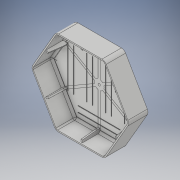
# Autodesk Inventor part: Base v5 - 175
Saved by Autodesk Inventor 2019 (Build 230136000, 136)
## iProperties
Created: 2021-07-14
Part Number: Base v5 - 175
Material: Generic
Document SubType Name: Modeling
Designer: Lix
Density: 1 g/cm^3
Appearance: Default
Author: Lix
## iProperties of the stored document Base v6 - 175 - thicker wall_3DPrint.ipt
Created: 2021-08-11
Part Number: Base v6 - 175 - thicker wall_3DPrint
Material: Generic
Document SubType Name: Modeling
Designer: Lix
Density: 1 g/cm^3
Appearance: Default
Author: Lix
Autodesk Inventor part; units mm, degrees
sketch "Sketch1" plane through (0, 0, 0) normal (0, 0, 1) x (1, 0, 0)
  line L0 (50.5181, -87.5) -> (-50.5181, -87.5)
  line L1 (-50.5181, -87.5) -> (-101.0363, 0)
  line L2 (-101.0363, 0) -> (-50.5181, 87.5)
  line L3 (-50.5181, 87.5) -> (50.5181, 87.5)
  line L4 (50.5181, 87.5) -> (101.0363, 0)
  line L5 (101.0363, 0) -> (50.5181, -87.5)
  point P0 (0, 0)
  point P1 (0, 0)
  point P2 (0, 0)
  dimension "d0" = 175
  constraints: 12 end point, 2 coincident, 1 horizontal, 13 other
  measures "d0" distance between parallel lines of L5 L2
extrude "Extrusion1" add sketch "Sketch1" along normal blind 40
shell "Shell1" thickness 2.5 removed faces 1 at (16.8394, -29.1667, 40) ; own thickness 1 on faces at (16.8394, -29.1667, 0)
sketch "Sketch11" plane through (-49.0748, -85, 1) normal (0, 0, 1) x (1, 0, 0)
  line L0 (-9.4252, 85) -> (107.5748, 85) construction
  line L1 (6.7369, 14.5052) -> (91.4127, 14.5052)
  line L2 (91.4127, 14.5052) -> (91.4127, 25.4948)
  line L3 (91.4127, 25.4948) -> (6.7369, 25.4948)
  line L4 (6.7369, 25.4948) -> (6.7369, 14.5052)
  line L5 (6.7369, 14.5052) -> (91.4127, 25.4948) construction
  line L6 (91.4127, 14.5052) -> (6.7369, 25.4948) construction
  line L7 (49.0748, 20) -> (49.0748, 150) construction
  line L8 (6.7369, 144.5052) -> (91.4127, 144.5052)
  line L9 (91.4127, 144.5052) -> (91.4127, 155.4948)
  line L10 (91.4127, 155.4948) -> (6.7369, 155.4948)
  line L11 (6.7369, 155.4948) -> (6.7369, 144.5052)
  line L12 (6.7369, 144.5052) -> (91.4127, 155.4948) construction
  line L13 (91.4127, 144.5052) -> (6.7369, 155.4948) construction
  line L14 (5.7369, 156.4948) -> (92.4127, 156.4948)
  line L15 (92.4127, 156.4948) -> (92.4127, 143.5052)
  line L16 (92.4127, 143.5052) -> (5.7369, 143.5052)
  line L17 (5.7369, 143.5052) -> (5.7369, 156.4948)
  line L18 (92.4127, 13.5052) -> (5.7369, 13.5052)
  line L19 (5.7369, 13.5052) -> (5.7369, 26.4948)
  line L20 (5.7369, 26.4948) -> (92.4127, 26.4948)
  line L21 (92.4127, 26.4948) -> (92.4127, 13.5052)
  line L22 (92.4127, 155.5) -> (5.7369, 155.5)
  line L23 (5.7369, 155.5) -> (5.7369, 144.5)
  line L24 (5.7369, 144.5) -> (92.4127, 144.5)
  line L25 (92.4127, 144.5) -> (92.4127, 155.5)
  line L26 (92.4127, 25.5) -> (5.7369, 25.5)
  line L27 (5.7369, 25.5) -> (5.7369, 14.5)
  line L28 (5.7369, 14.5) -> (92.4127, 14.5)
  line L29 (92.4127, 14.5) -> (92.4127, 25.5)
  line L30 (-3.9252, 128.5) -> (-3.9252, 41.5)
  line L31 (-14.9252, 41.5) -> (-14.9252, 128.5)
  line L32 (-14.9252, 128.5) -> (-3.9252, 41.5) construction
  line L33 (-3.9252, 128.5) -> (-14.9252, 41.5) construction
  line L34 (147.2243, 85) -> (98.1495, 0) projected
  line L35 (0, 170) -> (98.1495, 0) construction
  line L36 (-14.9252, 128.5) -> (-15.9252, 128.5)
  line L37 (-15.9252, 128.5) -> (-15.9252, 41.5)
  line L38 (-15.9252, 41.5) -> (-14.9252, 41.5)
  line L39 (-14.9252, 41.5) -> (-14.9252, 128.5)
  line L40 (-3.9252, 41.5) -> (-2.9252, 41.5)
  line L41 (-2.9252, 41.5) -> (-2.9252, 128.5)
  line L42 (-2.9252, 128.5) -> (-3.9252, 128.5)
  line L43 (-3.9252, 128.5) -> (-3.9252, 41.5)
  line L44 (36.0748, 41.5) -> (36.0748, 128.5)
  line L45 (35.0748, 41.5) -> (36.0748, 41.5)
  line L46 (36.0748, 128.5) -> (35.0748, 128.5)
  line L47 (35.0748, 128.5) -> (35.0748, 41.5)
  line L48 (35.0748, 128.5) -> (35.0748, 41.5)
  line L49 (24.0748, 41.5) -> (24.0748, 128.5)
  line L50 (24.0748, 128.5) -> (35.0748, 41.5) construction
  line L51 (24.0748, 41.5) -> (24.0748, 128.5)
  line L52 (24.0748, 128.5) -> (23.0748, 128.5)
  line L53 (23.0748, 128.5) -> (23.0748, 41.5)
  line L54 (23.0748, 41.5) -> (24.0748, 41.5)
  line L55 (35.0748, 128.5) -> (24.0748, 41.5) construction
  line L56 (75.0748, 41.5) -> (75.0748, 128.5)
  line L57 (74.0748, 41.5) -> (75.0748, 41.5)
  line L58 (75.0748, 128.5) -> (74.0748, 128.5)
  line L59 (74.0748, 128.5) -> (74.0748, 41.5)
  line L60 (74.0748, 128.5) -> (74.0748, 41.5)
  line L61 (63.0748, 41.5) -> (63.0748, 128.5)
  line L62 (63.0748, 128.5) -> (74.0748, 41.5) construction
  line L63 (63.0748, 41.5) -> (63.0748, 128.5)
  line L64 (63.0748, 128.5) -> (62.0748, 128.5)
  line L65 (62.0748, 128.5) -> (62.0748, 41.5)
  line L66 (62.0748, 41.5) -> (63.0748, 41.5)
  line L67 (74.0748, 128.5) -> (63.0748, 41.5) construction
  line L68 (114.0748, 41.5) -> (114.0748, 128.5)
  line L69 (113.0748, 41.5) -> (114.0748, 41.5)
  line L70 (114.0748, 128.5) -> (113.0748, 128.5)
  line L71 (113.0748, 128.5) -> (113.0748, 41.5)
  line L72 (113.0748, 128.5) -> (113.0748, 41.5)
  line L73 (102.0748, 41.5) -> (102.0748, 128.5)
  line L74 (102.0748, 128.5) -> (113.0748, 41.5) construction
  line L75 (102.0748, 41.5) -> (102.0748, 128.5)
  line L76 (102.0748, 128.5) -> (101.0748, 128.5)
  line L77 (101.0748, 128.5) -> (101.0748, 41.5)
  line L78 (101.0748, 41.5) -> (102.0748, 41.5)
  line L79 (113.0748, 128.5) -> (102.0748, 41.5) construction
  circle A0 centre (-41.4556, 85) radius 0.5
  circle A1 centre (-38.4556, 85) radius 0.5
  point P0 (49.0748, 85)
  point P1 (29.5748, 85)
  point P2 (68.5748, 85)
  point P3 (107.5748, 85)
  dimension "d147" = 130
  dimension "d151" = 1
  dimension "d156" = 1
  dimension "d157" = 11
  dimension "d158" = 87
  dimension "d167" = 117
  dimension "d168" = 1
  dimension "d169" = 87
  dimension "d170" = 1
  dimension "d171" = 87
  dimension "d174" = 39
  dimension "d179" = 1
  dimension "d180" = 1
  dimension "d181" = 3
  constraints: 158 end point, 17 parallel, 15 midpoint, 8 horizontal, 8 perpendicular, 4 point on line, 2 centre point, 2 equal length, 1 vertical, 75 other
  measures "d147" distance of L7.start L7.end
  measures "d151" distance between parallel lines of L10 L14
  measures "d156" distance between parallel lines of L1 L18
  measures "d157" distance of L30.end L31.start
  measures "d158" distance of L30.start L30.end
  measures "d167" distance of L0.start L0.end
  measures "d168" distance of L38.end L37.end
  measures "d169" distance of L37.end L36.end
  measures "d170" distance of L42.end L41.end
  measures "d171" distance of L41.end L40.end
  measures "d174" distance of L0.start point (29.575, 85)
  measures "d179" diameter of A0
  measures "d180" diameter of A1
  measures "d181" distance of A1.centre A0.centre
extrude "Extrusion9" add sketch "Sketch11" along normal blind 0.5 contours L14 L15 L22 L17 | L24 L15 L16 L17 | L18 L19 L28 L21 | L26 L19 L20 L21 | L42 L41 L40 L30 | L38 L37 L36 L31 | L45 L47 L46 L44 | L54 L53 L52 L49 | L57 L59 L58 L56 | L66 L65 L64 L61 | L69 L71 L70 L68 | L78 L77 L76 L73 | A0 | A1
ref_plane "Work Plane1" through (-25.2591, 43.75, 40) normal (0.8660254, 0.5, 0) x (0, 0, -1)
ref_plane "Work Plane2" through (-50.5181, 0, 0) normal (0, 1, 0) x (1, 0, 0)
ref_plane "Work Plane3" through (-25.2591, -43.75, 0) normal (-0.8660254, 0.5, 0) x (0, 0, 1)
sketch "Sketch12" plane through (-49.0748, -85, 1) normal (0, 0, 1) x (1, 0, 0)
  line L0 (98.1495, 0) -> (0, 0) projected
  line L1 (147.2243, 85) -> (98.1495, 0) projected
  line L2 (98.1495, 170) -> (147.2243, 85) projected
  line L3 (0, 170) -> (98.1495, 170) projected
  line L4 (-49.0748, 85) -> (0, 170) projected
  line L5 (0, 0) -> (-49.0748, 85) projected
  point P0 (49.0748, 85)
sketch "Sketch4" plane through (-49.0748, -85, 1) normal (0, 0, 1) x (1, 0, 0)
  line L0 (98.1495, 0) -> (0, 0) projected
  line L1 (147.2243, 85) -> (98.1495, 0) projected
  line L2 (98.1495, 170) -> (147.2243, 85) projected
  line L3 (0, 170) -> (98.1495, 170) projected
  line L4 (-49.0748, 85) -> (0, 170) projected
  line L5 (0, 0) -> (-49.0748, 85) projected
  line L6 (-18.9944, 127.1007) -> (2.8868, 165)
  line L7 (2.8868, 165) -> (46.6491, 165)
  line L8 (98.1495, 170) -> (0, 0) construction
  arc A0 (46.6491, 94.7014) -> (41.886, 91.9514) centre (49.0748, 85) ccw
  line L9 (-18.9944, 127.1007) -> (41.886, 91.9514)
  line L10 (46.6491, 165) -> (46.6491, 94.7014)
  circle A1 centre (49.0748, 85) radius 2.5
  arc A2 (39.4603, 87.75) -> (39.4603, 82.25) centre (49.0748, 85) ccw
  line L11 (-21.4201, 122.8993) -> (39.4603, 87.75)
  line L12 (-21.4201, 47.1007) -> (39.4603, 82.25)
  line L13 (-21.4201, 47.1007) -> (-43.3013, 85)
  line L14 (-43.3013, 85) -> (-21.4201, 122.8993)
  arc A3 (41.886, 78.0486) -> (46.6491, 75.2986) centre (49.0748, 85) ccw
  line L15 (-18.9944, 42.8993) -> (41.886, 78.0486)
  line L16 (46.6491, 5) -> (46.6491, 75.2986)
  line L17 (46.6491, 5) -> (2.8868, 5)
  line L18 (2.8868, 5) -> (-18.9944, 42.8993)
  arc A4 (51.5004, 75.2986) -> (56.2636, 78.0486) centre (49.0748, 85) ccw
  line L19 (51.5004, 5) -> (51.5004, 75.2986)
  line L20 (117.144, 42.8993) -> (56.2636, 78.0486)
  line L21 (117.144, 42.8993) -> (95.2628, 5)
  line L22 (95.2628, 5) -> (51.5004, 5)
  arc A5 (58.6892, 82.25) -> (58.6892, 87.75) centre (49.0748, 85) ccw
  line L23 (119.5696, 47.1007) -> (58.6892, 82.25)
  line L24 (119.5696, 122.8993) -> (58.6892, 87.75)
  line L25 (119.5696, 122.8993) -> (141.4508, 85)
  line L26 (141.4508, 85) -> (119.5696, 47.1007)
  arc A6 (56.2636, 91.9514) -> (51.5004, 94.7014) centre (49.0748, 85) ccw
  line L27 (117.144, 127.1007) -> (56.2636, 91.9514)
  line L28 (51.5004, 165) -> (51.5004, 94.7014)
  line L29 (51.5004, 165) -> (95.2628, 165)
  line L30 (95.2628, 165) -> (117.144, 127.1007)
  point P0 (-49.0748, 85)
  point P1 (0, 0)
  point P2 (98.1495, 0)
  point P3 (147.2243, 85)
  point P4 (98.1495, 170)
  dimension "d37" = 5
  dimension "d44" = 10
  dimension "d45" = 60
  dimension "d46" = 90
  dimension "d47" = 90
  dimension "d52" = 5.5
  dimension "d55" = 5
  dimension "d72" = 360
  constraints: 50 end point, 12 point on circle, 7 centre point, 2 coincident, 2 equal length, 1 midpoint, 73 other
  measures "d37" distance between parallel lines of L3 L7
  measures "d44" radius of A0
  measures "d45" angle of L10 L9
  measures "d46" angle of L9 L6
  measures "d47" angle of L10 L7
  measures "d52" distance of L10.end L9.end
  measures "d55" diameter of A1
extrude "Extrusion5" cut sketch "Sketch4" against normal blind 0.01 contours L6 L7 L10 A0 L9 | A1 | A2 L12 L13 L14 L11 | A3 L16 L17 L18 L15 | A4 L20 L21 L22 L19 | A5 L24 L25 L26 L23 | A6 L28 L29 L30 L27
sketch "Sketch8" plane through (-49.0748, -85, 1) normal (0, 0, 1) x (1, 0, 0)
  line L0 (98.1495, 0) -> (0, 0) projected
  line L1 (147.2243, 85) -> (98.1495, 0) projected
  line L2 (98.1495, 170) -> (147.2243, 85) projected
  line L3 (0, 170) -> (98.1495, 170) projected
  line L4 (-49.0748, 85) -> (0, 170) projected
  line L5 (0, 0) -> (-49.0748, 85) projected
  line L6 (47.5748, 162) -> (50.5748, 162)
  line L7 (50.5748, 162) -> (50.5748, 170)
  line L8 (50.5748, 170) -> (47.5748, 170)
  line L9 (47.5748, 170) -> (47.5748, 162)
  line L10 (0, 170) -> (98.1495, 170) projected
  line L11 (49.0748, 86) -> (49.0748, 170)
  point P0 (49.0748, 85)
  dimension "d57" = 3
  dimension "d58" = 8
  constraints: 10 end point, 2 midpoint, 2 parallel, 1 coincident, 1 collinear, 1 horizontal, 1 perpendicular, 1 vertical
  measures "d57" distance of L6.start L6.end
  measures "d58" distance of L6.end L7.end
extrude "Extrusion6" add sketch "Sketch8" along normal blind 36 contours L7 L6 L11 L3 | L3 L11 L6 L9
sketch "Sketch9" plane through (1.5, 77, 1) normal (1, 0, 0) x (0, 0, -1)
  line L0 (0, 0) -> (0, 8) projected
  line L1 (0, 0) -> (-36, 0) projected
  line L2 (-36, 8) -> (-36, 0) projected
  line L3 (0, 8) -> (-36, 8) projected
  line L4 (-36, 8) -> (-36, 0) projected
  line L5 (-36, 0) -> (-6, 0)
  line L6 (0, 0) -> (-36, 0) projected
  line L7 (-6, 0) -> (-36, 3)
  line L8 (-36, 3) -> (-36, 0)
  point P0 (1, -77)
  point P1 (-36, 8)
  dimension "d77" = 3
  dimension "d78" = 30
  constraints: 6 end point, 3 point on line, 1 collinear, 1 perpendicular
  measures "d77" distance of L7.end L5.start
  measures "d78" distance of L5.start L5.end
extrude "Extrusion8" cut sketch "Sketch9" against normal blind 20 contours L1 L2 L7
pattern_circular "Circular Pattern1" count 6 over 360 about axis through (0, 0, 1) along (0, 0, -1) of "Extrusion6", "Extrusion8"
fillet "Fillet1" radius 4 18 edges at (-25.2874, -85, 1) (25.2874, -85, 1) (-86.2559, -20.6005, 1) (-60.9685, -64.3995, 1) (60.9685, -64.3995, 1) (86.2559, -20.6005, 1) (86.2559, 20.6005, 1) (60.9685, 64.3995, 1) (25.2874, 85, 1) (-25.2874, 85, 1) (-60.9685, 64.3995, 1) (-86.2559, 20.6005, 1) (-98.1495, 0, 20.5) (-49.0748, 85, 20.5) (49.0748, 85, 20.5) (98.1495, 0, 20.5) (49.0748, -85, 20.5) (-49.0748, -85, 20.5)
fillet "Fillet2" radius 10 6 edges at (101.0363, 0, 20) (50.5181, 87.5, 20) (-50.5181, 87.5, 20) (50.5181, -87.5, 20) (-101.0363, 0, 20) (-50.5181, -87.5, 20)
fillet "Fillet4" radius 2 5 edges at (-7.1888, 6.9514, 0.995) (-2.4257, 9.7014, 0.995) (-2.4257, 80, 0.995) (-46.188, 80, 0.995) (-68.0692, 42.1007, 0.995)
sketch "Sketch5" plane through (-44.7446, 87.5, 0) normal (0, 1, 0) x (1, 0, 0)
  line L0 (0, 0) -> (89.4893, 0) projected
  line L1 (0, -40) -> (0, 0) projected
  point P0 (44.7446, 0)
  point P1 (44.7446, -20)
  point P2 (44.7446, 0)
  point P3 (0, -20)
  constraints: 2 midpoint, 1 horizontal alignment, 1 vertical alignment
sketch "Sketch6" plane through (53.4049, 82.5, 40) normal (0.8660254, 0.5, 0) x (0, 0, -1)
  line L0 (40, 8.6603) -> (0, 8.6603) projected
  point P0 (40, -44.7446)
  point P1 (20, -44.7446)
  point P2 (20, 8.6603)
  constraints: 1 horizontal alignment, 1 midpoint, 1 vertical alignment
sketch "Sketch7" plane through (53.4049, -82.5, 40) normal (0.8660254, -0.5, 0) x (0, 0, -1)
  line L0 (0, -8.6603) -> (40, -8.6603) projected
  point P0 (40, 44.7446)
  point P1 (20, 44.7446)
  point P2 (20, -8.6603)
  constraints: 1 horizontal alignment, 1 midpoint, 1 vertical alignment
sketch "Sketch13" plane through (0, 0, 40) normal (0, 0, 1) x (1, 0, 0)
  line L0 (-66.25, -43.5) -> (-55.25, -43.5) projected
  line L1 (-55.25, -43.5) -> (-55.25, 43.5) projected
  line L2 (-55.25, 43.5) -> (-66.25, 43.5) projected
  line L3 (-66.25, 43.5) -> (-66.25, -43.5) projected
  line L4 (-25.75, -43.5) -> (-14.75, -43.5) projected
  line L5 (-14.75, -43.5) -> (-14.75, 43.5) projected
  line L6 (-14.75, 43.5) -> (-25.75, 43.5) projected
  line L7 (-25.75, 43.5) -> (-25.75, -43.5) projected
  line L8 (-43.5, 59.5) -> (43.5, 59.5) projected
  line L9 (43.5, 59.5) -> (43.5, 70.5) projected
  line L10 (43.5, 70.5) -> (-43.5, 70.5) projected
  line L11 (-43.5, 70.5) -> (-43.5, 59.5) projected
  line L12 (14.75, -43.5) -> (25.75, -43.5) projected
  line L13 (25.75, -43.5) -> (25.75, 43.5) projected
  line L14 (25.75, 43.5) -> (14.75, 43.5) projected
  line L15 (14.75, 43.5) -> (14.75, -43.5) projected
  line L16 (55.25, -43.5) -> (66.25, -43.5) projected
  line L17 (66.25, -43.5) -> (66.25, 43.5) projected
  line L18 (66.25, 43.5) -> (55.25, 43.5) projected
  line L19 (55.25, 43.5) -> (55.25, -43.5) projected
  line L20 (-43.5, -70.5) -> (43.5, -70.5) projected
  line L21 (43.5, -70.5) -> (43.5, -59.5) projected
  line L22 (43.5, -59.5) -> (-43.5, -59.5) projected
  line L23 (-43.5, -59.5) -> (-43.5, -70.5) projected
  arc A0 (-53.4049, -82.5) -> (-44.7446, -87.5) centre (-44.7446, -77.5) ccw projected
  line L24 (-44.7446, -87.5) -> (44.7446, -87.5) projected
  arc A1 (44.7446, -87.5) -> (53.4049, -82.5) centre (44.7446, -77.5) ccw projected
  line L25 (53.4049, -82.5) -> (98.1495, -5) projected
  arc A2 (98.1495, -5) -> (98.1495, 5) centre (89.4893, 0) ccw projected
  line L26 (98.1495, 5) -> (53.4049, 82.5) projected
  arc A3 (53.4049, 82.5) -> (44.7446, 87.5) centre (44.7446, 77.5) ccw projected
  line L27 (44.7446, 87.5) -> (-44.7446, 87.5) projected
  arc A4 (-44.7446, 87.5) -> (-53.4049, 82.5) centre (-44.7446, 77.5) ccw projected
  line L28 (-53.4049, 82.5) -> (-98.1495, 5) projected
  arc A5 (-98.1495, 5) -> (-98.1495, -5) centre (-89.4893, 0) ccw projected
  line L29 (-98.1495, -5) -> (-53.4049, -82.5) projected
  line L30 (-50.2295, -83) -> (-96.9948, -2) projected
  arc A6 (-96.9948, 2) -> (-96.9948, -2) centre (-93.5307, 0) ccw projected
  line L31 (-96.9948, 2) -> (-50.2295, 83) projected
  arc A7 (-46.7654, 85) -> (-50.2295, 83) centre (-46.7654, 81) ccw projected
  line L32 (-46.7654, 85) -> (46.7654, 85) projected
  arc A8 (50.2295, 83) -> (46.7654, 85) centre (46.7654, 81) ccw projected
  line L33 (50.2295, 83) -> (96.9948, 2) projected
  arc A9 (96.9948, -2) -> (96.9948, 2) centre (93.5307, 0) ccw projected
  line L34 (96.9948, -2) -> (50.2295, -83) projected
  arc A10 (46.7654, -85) -> (50.2295, -83) centre (46.7654, -81) ccw projected
  line L35 (46.7654, -85) -> (-46.7654, -85) projected
  arc A11 (-50.2295, -83) -> (-46.7654, -85) centre (-46.7654, -81) ccw projected
  line L36 (1.5, -80) -> (-1.5, -80) projected
  line L37 (-1.5, -80) -> (-1.5, -85) projected
  line L38 (1.5, -85) -> (1.5, -80) projected
  line L39 (-68.532, -41.299) -> (-70.032, -38.701) projected
  line L40 (-70.032, -38.701) -> (-74.3622, -41.201) projected
  line L41 (-72.8622, -43.799) -> (-68.532, -41.299) projected
  line L42 (-65.934, -39.799) -> (-68.532, -41.299) projected
  line L43 (-67.434, -37.201) -> (-65.934, -39.799) projected
  line L44 (-70.032, -38.701) -> (-67.434, -37.201) projected
  line L45 (-68.532, -41.299) -> (-70.032, -38.701) projected
  line L46 (1.5, -77) -> (1.5, -80) projected
  line L47 (-1.5, -77) -> (1.5, -77) projected
  line L48 (-1.5, -80) -> (-1.5, -77) projected
  line L49 (1.5, -80) -> (-1.5, -80) projected
  line L50 (-70.032, 38.701) -> (-68.532, 41.299) projected
  line L51 (-68.532, 41.299) -> (-72.8622, 43.799) projected
  line L52 (-74.3622, 41.201) -> (-70.032, 38.701) projected
  line L53 (-67.434, 37.201) -> (-70.032, 38.701) projected
  line L54 (-65.934, 39.799) -> (-67.434, 37.201) projected
  line L55 (-68.532, 41.299) -> (-65.934, 39.799) projected
  line L56 (-70.032, 38.701) -> (-68.532, 41.299) projected
  line L57 (-1.5, 80) -> (1.5, 80) projected
  line L58 (1.5, 80) -> (1.5, 85) projected
  line L59 (-1.5, 85) -> (1.5, 85) projected
  line L60 (-1.5, 85) -> (-1.5, 80) projected
  line L61 (-1.5, 77) -> (-1.5, 80) projected
  line L62 (1.5, 77) -> (-1.5, 77) projected
  line L63 (1.5, 80) -> (1.5, 77) projected
  line L64 (-1.5, 80) -> (1.5, 80) projected
  line L65 (68.532, 41.299) -> (70.032, 38.701) projected
  line L66 (70.032, 38.701) -> (74.3622, 41.201) projected
  line L67 (72.8622, 43.799) -> (74.3622, 41.201) projected
  line L68 (72.8622, 43.799) -> (68.532, 41.299) projected
  line L69 (65.934, 39.799) -> (68.532, 41.299) projected
  line L70 (67.434, 37.201) -> (65.934, 39.799) projected
  line L71 (70.032, 38.701) -> (67.434, 37.201) projected
  line L72 (68.532, 41.299) -> (70.032, 38.701) projected
  line L73 (70.032, -38.701) -> (68.532, -41.299) projected
  line L74 (68.532, -41.299) -> (72.8622, -43.799) projected
  line L75 (74.3622, -41.201) -> (70.032, -38.701) projected
  line L76 (67.434, -37.201) -> (70.032, -38.701) projected
  line L77 (65.934, -39.799) -> (67.434, -37.201) projected
  line L78 (68.532, -41.299) -> (65.934, -39.799) projected
  line L79 (70.032, -38.701) -> (68.532, -41.299) projected
  line L80 (74.3622, -41.201) -> (72.8622, -43.799) projected
  line L81 (-74.3622, 41.201) -> (-72.8622, 43.799) projected
  line L82 (-72.8622, -43.799) -> (-74.3622, -41.201) projected
  line L83 (1.5, -85) -> (-1.5, -85) projected
  point P0 (0, 0)
body "Solid1"
